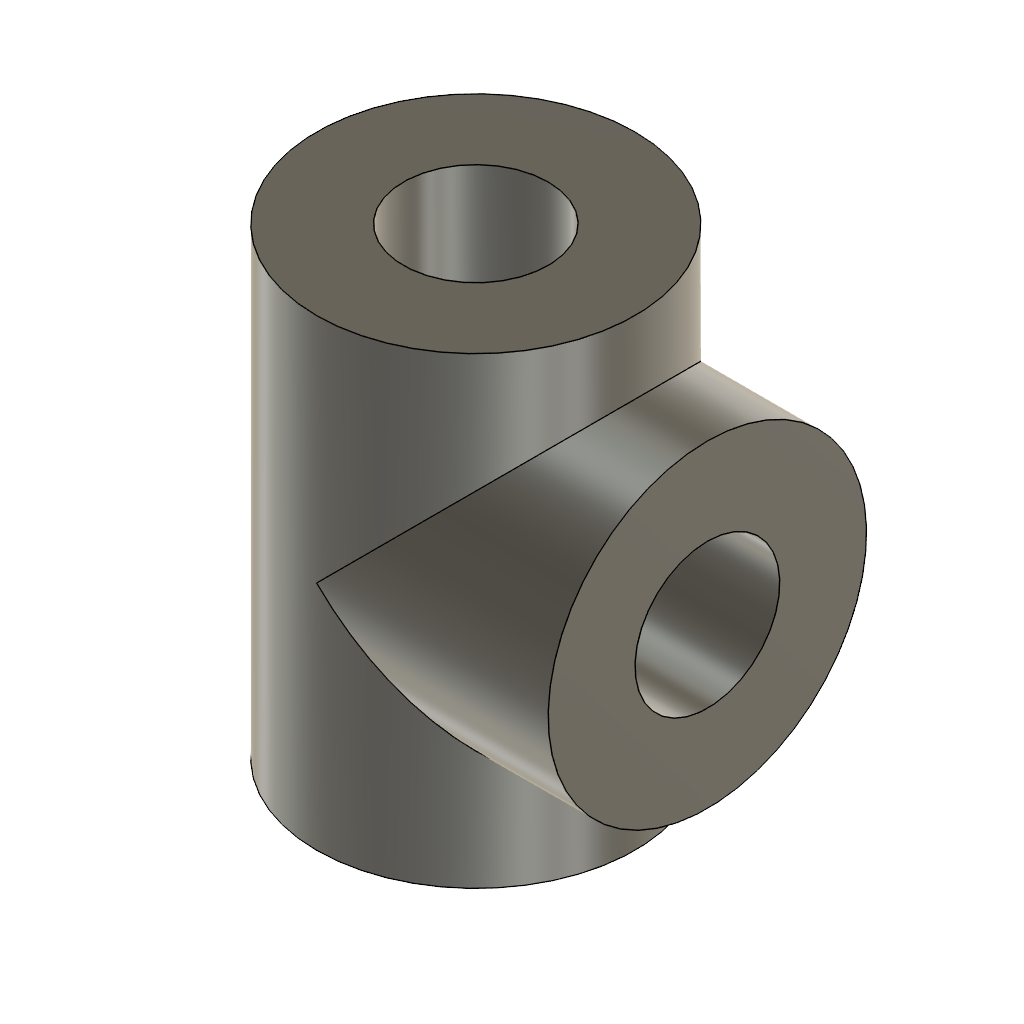
02 - T-SHAPE STANDARD EXTERNAL INVOLUTE MITER BEVEL GEAR CONNECTOR (Autodesk Fusion 360 design; units mm, degrees)
Autodesk Fusion 360 part; units mm, degrees
note: some values were not read from the file. Chosen so that the rebuilt part matches the saved one: which face or edge a step refers to; which pieces of a blend or face edit are solid. Set by a fixed rule: which sketch regions a step uses.
sketch "Sketch1" plane through (0, 0, 0) normal (1, 0, 0) x (0, 1, 0) in component "01 - T-SHAPE STANDARD EXTERNAL INVOLUTE MITER BEVEL GEAR CONNECTOR"
  circle A0 centre (0, 0) radius 11
  line L0 (0, 0) -> (0, 11)
  circle A1 centre (0, 0) radius 5
  dimension "d1" = 22
  dimension "d19" = 10
  constraint coincident A0.centre L0.start
  constraint coincident A0 L0.end
  constraint vertical L0
  measures "d1" diameter of A0
  measures "d19" diameter of A1
extrude "Extrude1" add sketch "Sketch1" along normal blind 16 and the other way blind 16 contours A0 | A1 in component "01 - T-SHAPE STANDARD EXTERNAL INVOLUTE MITER BEVEL GEAR CONNECTOR"
ref_plane "WorkPlane2" through (0, 0, 11) normal (0, 0, 1) x (1, 0, 0) in component "01 - T-SHAPE STANDARD EXTERNAL INVOLUTE MITER BEVEL GEAR CONNECTOR"
sketch "Sketch3" plane through (0, 0, 11) normal (0, 0, 1) x (1, 0, 0) in component "01 - T-SHAPE STANDARD EXTERNAL INVOLUTE MITER BEVEL GEAR CONNECTOR"
  circle A0 centre (0, 0) radius 11
  dimension "d13" = 22
  constraint coincident A0.centre origin
  measures "d13" diameter of A0
extrude "Extrude2" add sketch "Sketch3" along normal up to near side of body 1 in component "01 - T-SHAPE STANDARD EXTERNAL INVOLUTE MITER BEVEL GEAR CONNECTOR"
extrude "Extrude3" add 2 faces at (3.1924, -3.1463, 11) (-1.179, 5.1656, 11) along direction (0, 0, 1) blind 5 in component "01 - T-SHAPE STANDARD EXTERNAL INVOLUTE MITER BEVEL GEAR CONNECTOR"
shell "Shell1" thickness 6 removed faces 1 at (5.6593, -1.2423, 16) in component "01 - T-SHAPE STANDARD EXTERNAL INVOLUTE MITER BEVEL GEAR CONNECTOR"
hole "Hole1" at (16, 0, 0) direction (-1, 0, 0) diameter 10 depth 32 tip angle 180 in component "01 - T-SHAPE STANDARD EXTERNAL INVOLUTE MITER BEVEL GEAR CONNECTOR"
component "01 - T-SHAPE STANDARD EXTERNAL INVOLUTE MITER BEVEL GEAR CONNECTOR" placed x (0, 0, -1) y (0, 1, 0) z (1, 0, 0) at (-2.3743, 0, 2.3743)
named bodies: "01 - T-SHAPE STANDARD EXTERNAL INVOLUTE MITER BEVEL GEAR CONNECTOR"
